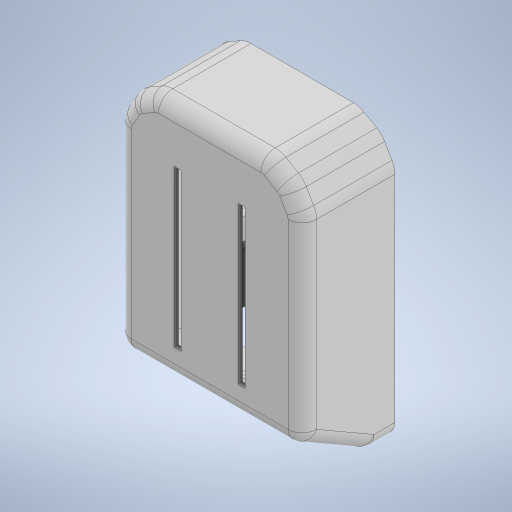
# Autodesk Inventor part: Terminal
Saved by Autodesk Inventor 2024 (Build 280153000, 153)
## iProperties
Created: 2026-05-14
Part Number: Terminal
Material: Generic
Document SubType Name: Modeling
Designer: janst
Density: 1 g/cm^3
Appearance: Default
Author: janst
Autodesk Inventor part; units mm, degrees
ref_plane "YZ Plane" through (0, 0, 0) normal (1, 0, 0) x (0, 1, 0)
ref_plane "XZ Plane" through (0, 0, 0) normal (0, 1, 0) x (-1, 0, 0)
ref_plane "XY Plane" through (0, 0, 0) normal (0, 0, 1) x (1, 0, 0)
sketch "Sketch1" plane through (0, 0, 0) normal (1, 0, 0) x (0, 1, 0)
  line L0 (200, 65) -> (37.5278, 65)
  line L1 (37.5278, 65) -> (0, 0)
  line L2 (0, 0) -> (200, 0)
  line L3 (200, 0) -> (200, 65)
  line L4 (10, 17.3205) -> (10, 0)
  dimension "d0" = 60
  dimension "d1" = 200
  dimension "d2" = 65
  dimension "d18" = 10
  constraints: 10 end point, 2 horizontal, 2 point on line, 1 coincident, 1 perpendicular, 1 vertical
  measures "d0" angle of L2 L1
  measures "d1" distance of L1.end L2.end
  measures "d2" distance of L2.end L0.start
  measures "d18" distance from line of L4 point (0, 0)
extrude "Extrusion1" add sketch "Sketch1" along normal blind 130 contours L3 L2 L4 L1 L0
sketch "Sketch2" plane through (0, 37.5278, 65) normal (0, 0, 1) x (1, 0, 0)
  line L0 (0, 162.4722) -> (0, 0) projected
  line L1 (0, 0) -> (130, 0) projected
  line L2 (130, 162.4722) -> (130, 0) projected
  line L3 (0, 162.4722) -> (130, 162.4722) projected
  line L4 (0, 137.4722) -> (9.1506, 153.3216)
  line L5 (9.1506, 153.3216) -> (25, 162.4722)
  line L6 (130, 137.4722) -> (120.8494, 153.3216)
  line L7 (120.8494, 153.3216) -> (105, 162.4722)
  point P0 (0, -37.5278)
  dimension "d5" = 25
  dimension "d6" = 30
  dimension "d7" = 30
  dimension "d8" = 25
  dimension "d9" = 30
  dimension "d10" = 30
  dimension "d11" = 25
  dimension "d12" = 25
  constraints: 8 end point, 4 point on line, 1 perpendicular
  measures "d5" distance from line of L3 L4.start
  measures "d6" angle of L0 L4
  measures "d7" angle of L3 L5
  measures "d8" distance from line of L0 L5.end
  measures "d9" angle of L2 L6
  measures "d10" angle of L3 L7
  measures "d11" distance from line of L3 L6.start
  measures "d12" distance from line of L2 L7.end
extrude "Extrusion2" cut sketch "Sketch2" against normal blind 130 contours L3 L5 L4 L0 | L3 L2 L6 L7
fillet "Fillet1" radius 10 13 edges at (112.9247, 195.4247, 65) (65, 200, 65) (17.0753, 195.4247, 65) (4.5753, 182.9247, 65) (0, 106.2639, 65) (130, 106.2639, 65) (125.4247, 182.9247, 65) (0, 23.7639, 41.1603) (65, 37.5278, 65) (130, 23.7639, 41.1603) (65, 10, 17.3205) (130, 10, 8.6603) (0, 10, 8.6603)
shell "Shell1" thickness 3 removed faces 1 at (86.6667, 123.3333, 0)
fillet "Fillet2" radius 15 12 edges at (2.9289, 174.2152, 62.0711) (0, 175, 27.5) (11.2948, 188.7052, 62.0711) (9.1506, 190.8494, 27.5) (25.7848, 197.0711, 62.0711) (25, 200, 27.5) (104.2152, 197.0711, 62.0711) (105, 200, 27.5) (118.7052, 188.7052, 62.0711) (120.8494, 190.8494, 27.5) (127.0711, 174.2152, 62.0711) (130, 175, 27.5)
sketch "Sketch3" plane through (10, 43.3013, 65) normal (0, 0, 1) x (1, 0, 0)
  line L0 (75, 10) -> (80, 10)
  line L1 (80, 10) -> (80, 120)
  line L2 (80, 120) -> (75, 120)
  line L3 (75, 120) -> (75, 10)
  line L4 (75, 10) -> (80, 120) construction
  line L5 (80, 10) -> (75, 120) construction
  line L6 (30, 10) -> (35, 10)
  line L7 (35, 10) -> (35, 120)
  line L8 (35, 120) -> (30, 120)
  line L9 (30, 120) -> (30, 10)
  line L10 (30, 10) -> (35, 120) construction
  line L11 (35, 10) -> (30, 120) construction
  arc A0 (110, 127.6795) -> (109.3301, 130.1795) centre (105, 127.6795) ccw projected
  line L12 (104.1987, 139.0673) -> (109.3301, 130.1795) projected
  arc A1 (104.1987, 139.0673) -> (102.3686, 140.8975) centre (99.8686, 136.5673) ccw projected
  line L13 (93.4808, 146.0289) -> (102.3686, 140.8975) projected
  arc A2 (93.4808, 146.0289) -> (90.9808, 146.6987) centre (90.9808, 141.6987) ccw projected
  line L14 (19.0192, 146.6987) -> (90.9808, 146.6987) projected
  arc A3 (19.0192, 146.6987) -> (16.5192, 146.0289) centre (19.0192, 141.6987) ccw projected
  line L15 (7.6314, 140.8975) -> (16.5192, 146.0289) projected
  arc A4 (7.6314, 140.8975) -> (5.8013, 139.0673) centre (10.1314, 136.5673) ccw projected
  line L16 (0.6699, 130.1795) -> (5.8013, 139.0673) projected
  arc A5 (0.6699, 130.1795) -> (0, 127.6795) centre (5, 127.6795) ccw projected
  line L17 (0, 0) -> (0, 127.6795) projected
  line L18 (110, 0) -> (0, 0) projected
  line L19 (110, 127.6795) -> (110, 0) projected
  point P0 (-10, -43.3013)
  point P1 (77.5, 65)
  point P2 (32.5, 65)
  dimension "d19" = 5
  dimension "d20" = 110
  dimension "d21" = 110
  dimension "d22" = 5
  dimension "d23" = 30
  dimension "d24" = 30
  dimension "d25" = 10
  dimension "d26" = 10
  constraints: 24 end point, 4 midpoint, 4 parallel, 2 horizontal, 2 perpendicular
  measures "d19" distance of L0.start L0.end
  measures "d20" distance of L0.end L1.end
  measures "d21" distance of L8.end L6.start
  measures "d22" distance of L7.end L8.end
  measures "d23" distance between parallel lines of L19 L1
  measures "d24" distance between parallel lines of L17 L9
  measures "d25" distance between parallel lines of L18 L0
  measures "d26" distance between parallel lines of L18 L6
extrude "Extrusion3" cut sketch "Sketch3" against normal blind 130 contours L3 L2 L1 L0 | L9 L8 L7 L6
sketch "Sketch4" plane through (0, 0, 0) normal (-1, 0, 0) x (0, 0, 1)
  line L0 (0, 170.9808) -> (55, 170.9808) projected
  line L1 (0, 20) -> (0, 170.9808) projected
  line L2 (14.641, 20) -> (0, 20) projected
  line L3 (55, 43.3013) -> (14.641, 20) projected
  line L4 (55, 170.9808) -> (55, 43.3013) projected
  circle A0 centre (27.5, 145.9808) radius 5
  point P0 (0, 0)
  dimension "d29" = 10
  dimension "d30" = 25
  dimension "d31" = 27.5
  dimension "d32" = 55
  constraints: 1 centre point
  measures "d29" diameter of A0
  measures "d30" distance from line of L0 A0.centre
  measures "d31" distance from line of L4 A0.centre
  measures "d32" distance between parallel lines of L1 L4
extrude "Extrusion4" cut sketch "Sketch4" against normal up to surface (3 mm away) contours A0
sketch "Sketch5" plane through (10, 13.9378, 18.141) normal (0, 0.8660254, -0.5) x (1, 0, 0)
  line L0 (110, 0) -> (0, 0) projected
  line L1 (0, 0) -> (0, -46.6025) projected
  line L2 (0, -46.6025) -> (110, -46.6025) projected
  line L3 (110, -46.6025) -> (110, 0) projected
  line L4 (80, -40) -> (30, -40)
  line L5 (30, -40) -> (30, -5)
  line L6 (30, -5) -> (80, -5)
  line L7 (80, -5) -> (80, -40)
  line L8 (80, -40) -> (30, -5) construction
  line L9 (30, -40) -> (80, -5) construction
  point P0 (-10, 22.6795)
  point P1 (55, -22.5)
  dimension "d35" = 50
  dimension "d36" = 35
  dimension "d37" = 5
  dimension "d38" = 110
  dimension "d39" = 30
  constraints: 12 end point, 2 midpoint, 2 parallel, 1 horizontal, 1 perpendicular
  measures "d35" distance of L5.end L6.end
  measures "d36" distance of L4.end L5.end
  measures "d37" distance between parallel lines of L0 L6
  measures "d38" distance of L1.end L2.end
  measures "d39" distance between parallel lines of L3 L7
extrude "Extrusion5" cut sketch "Sketch5" against normal blind 2 contours L4 L5 L6 L7
sketch "Sketch6" plane through (120, 43.3013, 62) normal (0, 0, -1) x (-1, 0, 0)
  line L0 (75, 120) -> (80, 120) projected
  line L1 (80, 120) -> (80, 10) projected
  line L2 (80, 10) -> (75, 10) projected
  line L3 (75, 10) -> (75, 120) projected
  line L4 (30, 120) -> (35, 120) projected
  line L5 (35, 120) -> (35, 10) projected
  line L6 (35, 10) -> (30, 10) projected
  line L7 (30, 10) -> (30, 120) projected
  line L8 (17.6795, 146.6987) -> (6.4711, 140.2276) projected
  line L9 (6.4711, 140.2276) -> (0, 129.0192) projected
  line L10 (0, 129.0192) -> (0, 0) projected
  line L11 (0, 0) -> (110, 0) projected
  line L12 (110, 0) -> (110, 129.0192) projected
  line L13 (110, 129.0192) -> (103.5289, 140.2276) projected
  line L14 (103.5289, 140.2276) -> (92.3205, 146.6987) projected
  line L15 (92.3205, 146.6987) -> (17.6795, 146.6987) projected
  line L16 (67.5, 47.5) -> (62.5, 47.5)
  line L17 (62.5, 47.5) -> (62.5, 82.5)
  line L18 (62.5, 82.5) -> (67.5, 82.5)
  line L19 (67.5, 82.5) -> (67.5, 47.5)
  line L20 (67.5, 47.5) -> (62.5, 82.5) construction
  line L21 (62.5, 47.5) -> (67.5, 82.5) construction
  line L22 (47.5, 82.5) -> (42.5, 82.5)
  line L23 (42.5, 82.5) -> (42.5, 47.5)
  line L24 (42.5, 47.5) -> (47.5, 47.5)
  line L25 (47.5, 47.5) -> (47.5, 82.5)
  line L26 (47.5, 82.5) -> (42.5, 47.5) construction
  line L27 (42.5, 82.5) -> (47.5, 47.5) construction
  line L28 (35, 10) -> (30, 10) projected
  line L29 (80, 10) -> (75, 10) projected
  point P0 (120, -43.3013)
  point P1 (65, 65)
  point P2 (45, 65)
  point P3 (32.5, 10)
  point P4 (32.5, 10)
  point P5 (45, 47.5)
  point P6 (77.5, 10)
  point P7 (77.5, 10)
  point P8 (65, 47.5)
  dimension "d42" = 5
  dimension "d43" = 5
  dimension "d44" = 35
  dimension "d45" = 35
  dimension "d46" = 15
  dimension "d47" = 40
  dimension "d48" = 7.5
  dimension "d49" = 110
  dimension "d51" = 37.5
  dimension "d53" = 37.5
  constraints: 24 end point, 10 midpoint, 4 parallel, 2 horizontal, 2 perpendicular
  measures "d42" distance of L23.end L24.end
  measures "d43" distance of L16.start L16.end
  measures "d44" distance of L18.end L16.start
  measures "d45" distance of L22.end L23.end
  measures "d46" distance between parallel lines of L25 L17
  measures "d47" distance between parallel lines of L5 L3
  measures "d48" distance between parallel lines of L3 L19
  measures "d49" distance of L6.end L4.start
  measures "d51" vertical distance of point (32.5, 10) point (45, 47.5)
  measures "d53" vertical distance of point (77.5, 10) point (65, 47.5)
extrude "Extrusion6" add sketch "Sketch6" along normal blind 35 contours L16 L17 L18 L19 | L25 L24 L23 L22
equation "\"d7\" = d6"
equation "\"d8\" = d5"
equation "\"d10\" = d7"
equation "\"d11\" = d5"
equation "\"d12\" = d8"
equation "\"d21\" = d20"
equation "\"d22\" = d19"
equation "\"d24\" = d23"
equation "\"d26\" = d25"
equation "\"d31\" = 0.5 * d32"
equation "\"d39\" = -0.5 * d35 + 0.5 * d38"
equation "\"d43\" = d42"
equation "\"d45\" = d44"
equation "\"d48\" = -0.5 * d43 - 0.5 * d46 + 0.5 * d47 - 0.5 * d42"
equation "\"d51\" = -0.5 * d45 + 0.5 * d49"
equation "\"d53\" = d51"
body "Solid1"
